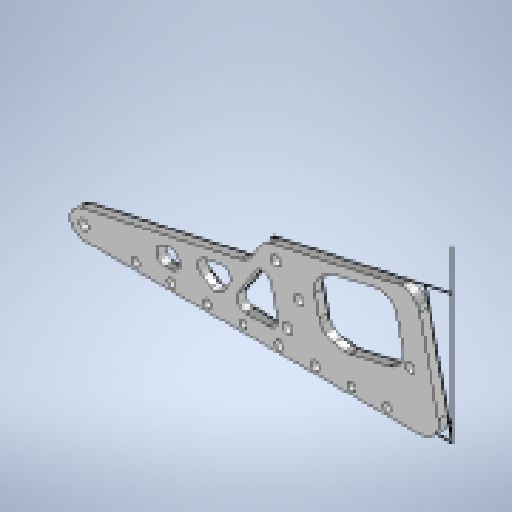
# Autodesk Inventor part: Uprights
Saved by Autodesk Inventor 2023.2 (Build 272271000, 271)
## iProperties
Created: 2024-01-11
Part Number: Uprights
Material: Aluminum 6061
Document SubType Name: Modeling
Designer: Nathan Cai
Mass: 19.8447 g
Surface Area: 66.3335 cm^2
Volume: 7.34987 cm^3
Density: 2.7 g/cm^3
Appearance: Aluminum - Flat
Slide_Offset: 1.875 in
Author: Nathan Cai
Autodesk Inventor part; units mm, degrees
ref_plane "YZ Plane" through (0, 0, 0) normal (1, 0, 0) x (0, 1, 0)
ref_plane "XZ Plane" through (0, 0, 0) normal (0, 1, 0) x (-1, 0, 0)
ref_plane "XY Plane" through (0, 0, 0) normal (0, 0, 1) x (1, 0, 0)
sketch "Sketch3" plane through (0, 0, 0) normal (0, 0, 1) x (1, 0, 0)
  line L0 (-48.8137, 10.438) -> (-52.9368, 29.0364) construction
  line L1 (-52.9368, 29.0364) -> (-59.1363, 27.662) construction
  line L2 (-59.1363, 27.662) -> (-55.0132, 9.0636) construction
  line L3 (-55.0132, 9.0636) -> (-48.8137, 10.438) construction
  line L4 (-48.8137, 10.438) -> (-59.1363, 27.662) construction
  line L5 (-52.9368, 29.0364) -> (-55.0132, 9.0636) construction
  circle A0 centre (-50.8753, 19.7372) radius 1.7526
  circle A1 centre (-59.1363, 27.662) radius 1.7526
  circle A2 centre (-55.0132, 9.0636) radius 1.7526
  line L6 (0, 0) -> (-127, 0)
  line L7 (0, 60.0769) -> (0, 0)
  line L8 (-44.6831, 6.4756) -> (-50.8679, 34.3732)
  line L9 (-50.8679, 34.3732) -> (-63.2669, 31.6244)
  line L10 (-63.2669, 31.6244) -> (-57.0821, 3.7268)
  line L11 (-57.0821, 3.7268) -> (-44.6831, 6.4756)
  line L12 (-44.6831, 6.4756) -> (-63.2669, 31.6244) construction
  line L13 (-50.8679, 34.3732) -> (-57.0821, 3.7268) construction
  line L14 (-50.1807, 31.2735) -> (-17.6334, 38.489)
  line L15 (-17.6334, 38.489) -> (-12.8231, 16.7909)
  line L16 (-12.8231, 16.7909) -> (-45.3703, 9.5753)
  line L17 (-45.3703, 9.5753) -> (-50.1807, 31.2735)
  line L18 (-47.081, 31.9607) -> (-42.2706, 10.2625)
  line L19 (-50.8679, 34.3732) -> (0, 45.6504)
  circle A3 centre (-127, 4.7625) radius 4.7625
  line L20 (-127, 0) -> (-127, 4.7625) construction
  line L21 (-128.0308, 9.4121) -> (-69.0937, 22.4782)
  line L22 (-79.3685, 6.35) -> (-63.2669, 31.6244)
  line L23 (-42.9578, 13.3622) -> (-33.7541, 12.1506)
  line L24 (-46.3938, 28.8609) -> (-38.5645, 33.8487)
  line L25 (-9.6463, 43.5118) -> (0, 0)
  circle A4 centre (-127, 4.7625) radius 1.7526
  line L26 (-111.125, 0) -> (-12.7, 0) construction
  line L27 (-12.7, 0) -> (-12.7, 4.7625) construction
  line L28 (-12.7, 4.7625) -> (-111.125, 4.7625) construction
  line L29 (-111.125, 4.7625) -> (-111.125, 0) construction
  line L30 (-12.7, 2.3812) -> (-111.125, 2.3812) construction
  circle A5 centre (-108.7437, 2.3812) radius 1.4732
  circle A6 centre (-96.0437, 2.3812) radius 1.4732
  circle A7 centre (-83.3438, 2.3812) radius 1.4732
  circle A8 centre (-70.6437, 2.3812) radius 1.4732
  circle A9 centre (-57.9438, 2.3812) radius 1.4732
  circle A10 centre (-45.2438, 2.3812) radius 1.4732
  circle A11 centre (-32.5438, 2.3812) radius 1.4732
  circle A12 centre (-19.8438, 2.3812) radius 1.4732
  circle A13 centre (-8.5171, 19.3715) radius 1.7526
  line L31 (-127.3436, 6.3124) -> (-67.1225, 19.6631)
  line L32 (-75.6039, 6.35) -> (-62.295, 27.2407)
  line L33 (0, 6.35) -> (-127, 6.35)
  line L34 (-79.3685, 6.35) -> (-91.7097, 14.2122)
  line L35 (-85.2776, 6.35) -> (-96.0934, 13.2404)
  point P0 (-53.975, 19.05)
  point P1 (-53.975, 19.05)
  point P2 (-53.975, 19.05)
  point P3 (-45.3703, 9.5753)
  point P4 (-127, 0)
  point P5 (-122.9599, 7.2842)
  point P6 (-122.5099, 6.35)
  point P7 (-57.6637, 6.35)
  point P8 (-71.5062, 18.6912)
  dimension "d71" = 19.05
  dimension "d72" = 6.35
  dimension "d73" = 3.5052
  dimension "d74" = 3.5052
  dimension "d75" = 3.5052
  dimension "d76" = 127
  dimension "d77" = 19.05
  dimension "d78" = 12.5
  dimension "d91" = 12.7
  dimension "d92" = 28.575
  dimension "d93" = 53.975
  dimension "d94" = 33.3375
  dimension "d95" = 3.175
  dimension "d96" = 3.175
  dimension "d97" = 3.175
  dimension "d98" = 9.525
  dimension "d100" = 45
  dimension "d102" = 20
  dimension "d103" = 20
  dimension "d104" = 3.175
  dimension "d105" = 3.175
  dimension "d107" = 3.5052
  dimension "d108" = 98.425
  dimension "d109" = 4.7625
  dimension "d110" = 15.875
  dimension "d111" = 2.9464
  dimension "d112" = 2.3813
  dimension "d115" = 12.7
  dimension "d120" = 3.5052
  dimension "Slide_Offset" = 47.625
  dimension "d124" = 3.175
  dimension "d125" = 6.35
  dimension "d126" = 3.175
  dimension "d127" = 3.175
  constraints: 72 end point, 21 point on line, 14 centre point, 14 parallel, 9 midpoint, 7 perpendicular, 3 coincident, 3 horizontal, 2 point on circle, 2 tangent, 2 vertical, 14 other
  measures "d71" distance between parallel lines of L3 L1
  measures "d72" distance between parallel lines of L2 L0
  measures "d73" diameter of A0
  measures "d74" diameter of A1
  measures "d75" diameter of A2
  measures "d76" distance of L6.start L6.end
  measures "d77" distance from line of L6 point (-53.975, 19.05)
  measures "d78" angle of L6 L3
  measures "d91" distance between parallel lines of L10 L8
  measures "d92" distance between parallel lines of L11 L9
  measures "d93" distance from line of L7 point (-53.975, 19.05)
  measures "d94" distance between parallel lines of L17 L15
  measures "d95" distance between parallel lines of L9 L14
  measures "d96" distance between parallel lines of L11 L16
  measures "d97" distance between parallel lines of L17 L18
  measures "d98" diameter of A3
  measures "d100" angle of L10 L22
  measures "d102" angle of L14 L24
  measures "d103" angle of L16 L23
  measures "d104" distance from line of L14 L24.start
  measures "d105" distance from line of L16 L23.start
  measures "d107" diameter of A4
  measures "d108" distance of L28.end L27.end
  measures "d109" distance of L27.end L26.end
  measures "d110" distance between parallel lines of L20 L29
  measures "d111" diameter of A5
  measures "d112" distance from line of A5.centre L29
  measures "d115" distance of A5.centre A6.centre
  measures "d120" diameter of A13
  measures "Slide_Offset" distance from line of L2 A13.centre
  measures "d124" distance between parallel lines of L21 L31
  measures "d125" distance between parallel lines of L6 L33
  measures "d126" distance between parallel lines of L22 L32
  measures "d127" distance between parallel lines of L34 L35
extrude "Extrusion3" add sketch "Sketch3" along normal blind 3.175 contours L6 A3 L33 L10 L11 L25 | A3 L31 A4 L33 | L33 L11 L8 L16 L15 L14 L19 L25 | L21 L22 L31 A3 | L33 L10 L9 L8 L11 | L11 L10 L33 | A3 L33 A4 L31 | L22 L10 L32 L31 | L31 L34 L33 L35 | L31 L32 L33 L22 | L14 L18 L16 L8 | L14 L24 L18 | L18 L23 L16 | A13
fillet "Fillet5" radius 6.35 10 edges at (-69.0937, 22.4782, 1.5875) (-63.2669, 31.6244, 1.5875) (-17.6334, 38.489, 1.5875) (-12.8231, 16.7909, 1.5875) (-46.3938, 28.8609, 1.5875) (-38.5645, 33.8487, 1.5875) (-33.7541, 12.1506, 1.5875) (-42.9578, 13.3622, 1.5875) (-9.6463, 43.5118, 1.5875) (0, 0, 1.5875)
extrude "Extrusion4" cut sketch "Sketch3" along normal blind 3.175 contours A13
fillet "Fillet6" radius 3.175 10 edges at (-62.295, 27.2407, 1.5875) (-57.6637, 6.35, 1.5875) (-75.6039, 6.35, 1.5875) (-71.5062, 18.6912, 1.5875) (-91.7097, 14.2122, 1.5875) (-79.3685, 6.35, 1.5875) (-85.2776, 6.35, 1.5875) (-96.0934, 13.2404, 1.5875) (-122.9599, 7.2842, 1.5875) (-122.5099, 6.35, 1.5875)
equation "\"Angle_Mount\" = 105deg"
equation "\"Rail_Offset\" = 36.5125"
body "Solid3"
